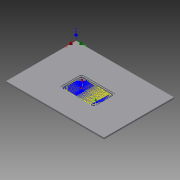
# Autodesk Inventor part: capac cu gaura 3
Saved by Autodesk Inventor 2015 SP1 (Build 190203100, 203)
## iProperties
Created: 2015-07-29
Part Number: capac cu gaura 3
Material: Generic
Document SubType Name: Modeling
Designer: ubik
Density: 1 g/cm^3
Appearance: Default
Author: ubik
Autodesk Inventor part; units mm, degrees
ref_plane "YZ Plane" through (0, 0, 0) normal (1, 0, 0) x (0, 1, 0)
ref_plane "XZ Plane" through (0, 0, 0) normal (0, 1, 0) x (-1, 0, 0)
ref_plane "XY Plane" through (0, 0, 0) normal (0, 0, 1) x (1, 0, 0)
sketch "Sketch1" plane through (0, 0, 0) normal (0, 0, 1) x (1, 0, 0)
  line L0 (0, 0) -> (560, 0)
  line L1 (560, 0) -> (560, 400)
  line L2 (560, 400) -> (0, 400)
  line L3 (0, 400) -> (0, 0)
  dimension "d0" = 560
  dimension "d1" = 400
  constraints: 8 end point, 2 parallel, 1 horizontal, 1 perpendicular
  measures "d0" distance of L2.end L1.end
  measures "d1" distance of L1.end L0.end
extrude "Extrusion1" add sketch "Sketch1" along normal blind 8
sketch "Sketch2" plane through (0, 0, 8) normal (0, 0, 1) x (1, 0, 0)
  line L0 (181.25, 250) -> (378.75, 250)
  line L1 (378.75, 250) -> (378.75, 124)
  line L2 (378.75, 124) -> (181.25, 124)
  line L3 (181.25, 124) -> (181.25, 250)
  line L4 (0, 400) -> (0, 0) projected
  line L5 (560, 400) -> (0, 400) projected
  line L6 (186.25, 245) -> (373.75, 245)
  line L7 (373.75, 245) -> (373.75, 129)
  line L8 (373.75, 129) -> (186.25, 129)
  line L9 (186.25, 129) -> (186.25, 245)
  dimension "cuva_width" = 197.5
  dimension "d5" = 126
  dimension "d6" = 181.25
  dimension "d7" = 150
  dimension "d8" = 5
  dimension "d9" = 5
  dimension "d10" = 5
  dimension "d11" = 5
  constraints: 16 end point, 4 parallel, 2 horizontal, 2 perpendicular
  measures "cuva_width" distance of L0.start L0.end
  measures "d5" distance of L2.end L0.start
  measures "d6" distance between parallel lines of L4 L3
  measures "d7" distance between parallel lines of L5 L0
  measures "d8" distance between parallel lines of L0 L6
  measures "d9" distance between parallel lines of L3 L9
  measures "d10" distance between parallel lines of L2 L8
  measures "d11" distance between parallel lines of L1 L7
extrude "Extrusion2" cut sketch "Sketch2" against normal blind 4
fillet "Fillet1" radius 12 4 edges at (181.25, 250, 6) (181.25, 124, 6) (378.75, 124, 6) (378.75, 250, 6)
sketch "Sketch3" plane through (0, 0, 8) normal (0, 0, 1) x (1, 0, 0)
  line L0 (186.25, 245) -> (186.25, 129) projected
  line L1 (186.25, 129) -> (373.75, 129) projected
  line L2 (373.75, 129) -> (373.75, 245) projected
  line L3 (373.75, 245) -> (186.25, 245) projected
  point P0 (0, 0)
extrude "Extrusion3" cut sketch "Sketch3" against normal blind 4
sketch "Sketch4" plane through (0, 0, 4) normal (0, 0, 1) x (1, 0, 0)
  arc A0 (378.75, 238) -> (366.75, 250) centre (366.75, 238) ccw projected
  line L0 (193.25, 250) -> (366.75, 250) projected
  arc A1 (193.25, 250) -> (181.25, 238) centre (193.25, 238) ccw projected
  line L1 (181.25, 136) -> (181.25, 238) projected
  arc A2 (181.25, 136) -> (193.25, 124) centre (193.25, 136) ccw projected
  line L2 (366.75, 124) -> (193.25, 124) projected
  arc A3 (366.75, 124) -> (378.75, 136) centre (366.75, 136) ccw projected
  line L3 (378.75, 238) -> (378.75, 136) projected
  line L4 (198.25, 245) -> (361.75, 245)
  line L5 (373.75, 233) -> (373.75, 141)
  line L6 (361.75, 129) -> (198.25, 129)
  line L7 (186.25, 141) -> (186.25, 233)
  arc A4 (198.25, 245) -> (186.25, 233) centre (198.25, 233) ccw
  arc A5 (186.25, 141) -> (198.25, 129) centre (198.25, 141) ccw
  arc A6 (373.75, 233) -> (361.75, 245) centre (361.75, 233) ccw
  arc A7 (361.75, 129) -> (373.75, 141) centre (361.75, 141) ccw
  point P0 (0, 0)
  dimension "d17" = 5
  dimension "d18" = 5
  dimension "d19" = 5
  dimension "d20" = 5
  dimension "d21" = 12
  constraints: 8 end point, 8 point on circle, 8 tangent, 4 centre point, 3 equal radius, 2 parallel, 1 horizontal, 1 perpendicular
  measures "d17" distance between parallel lines of L0 L4
  measures "d18" distance between parallel lines of L1 L7
  measures "d19" distance between parallel lines of L2 L6
  measures "d20" distance between parallel lines of L3 L5
  measures "d21" radius of A4
extrude "Extrusion4" cut sketch "Sketch4" against normal through all contours L4 A6 L5 A7 L6 A5 L7 A4
equation "\"d9\" = d8"
equation "\"d10\" = d8"
equation "\"d11\" = d8"
equation "\"d18\" = d17"
equation "\"d19\" = d17"
equation "\"d20\" = d17"
body "Solid1"
